Autodesk Fusion 360 part; units mm, degrees
note: some values were not read from the file. Set by a fixed rule: which sketch regions a step uses.
(part 2 of 4)
sketch "スケッチ25" plane through (0, 0, 3) normal (0, 0, 1) x (-1, 0, 0)
  line L0 (26.0567, 42.6737) -> (45.0073, 61.6244)
  line L1 (45.0073, 61.6244) -> (61.6244, 45.0073)
  line L2 (61.6244, 45.0073) -> (42.6737, 26.0567)
  arc A0 (42.6737, 26.0567) -> (26.0567, 42.6737) centre (0, 0) ccw
  line L3 (-36.2136, -34.4757) -> (-59.4233, -47.8758)
  line L4 (-59.4233, -47.8758) -> (-71.1733, -27.5242)
  line L5 (-71.1733, -27.5242) -> (-47.9636, -14.1241)
  arc A1 (-47.9636, -14.1241) -> (-36.2136, -34.4757) centre (0, 0) ccw
  arc A2 (-32.4242, -38.0614) -> (-21.7945, -45) centre (0, 0) ccw
  line L6 (-21.7945, -45) -> (-44.4423, -45)
  line L7 (-44.4423, -45) -> (-32.4242, -38.0614)
  line L8 (81.8683, -9) -> (73.6733, -23.1941)
  line L9 (73.6733, -23.1941) -> (49.1742, -9.0495)
  line L10 (49.1742, -9.0495) -> (75, -9)
  line L11 (75, -9) -> (81.8683, -9)
  line L12 (-42.6737, 26.0567) -> (-61.6244, 45.0073)
  line L13 (-61.6244, 45.0073) -> (-45.0073, 61.6244)
  line L14 (-45.0073, 61.6244) -> (-26.0567, 42.6737)
  arc A3 (-26.0567, 42.6737) -> (-42.6737, 26.0567) centre (0, 0) ccw
  line L15 (47.9636, -14.1241) -> (71.1733, -27.5242)
  line L16 (71.1733, -27.5242) -> (59.4233, -47.8758)
  line L17 (59.4233, -47.8758) -> (36.2136, -34.4757)
  arc A4 (36.2136, -34.4757) -> (47.9636, -14.1241) centre (0, 0) ccw
  line L18 (-81.8759, -8.9868) -> (-49.1742, -9.0495)
  line L19 (-49.1742, -9.0495) -> (-73.6733, -23.1941)
  line L20 (-73.6733, -23.1941) -> (-81.8759, -8.9868)
  line L21 (32.4242, -38.0614) -> (44.4423, -45)
  line L22 (44.4423, -45) -> (21.7945, -45)
  arc A5 (21.7945, -45) -> (32.4242, -38.0614) centre (0, 0) ccw
  arc A6 (44.8219, 4) -> (33.996, 29.4834) centre (0, 0) ccw
  line L23 (44.8219, 4) -> (98.9192, 4)
  arc A7 (98.9192, -4) -> (98.9192, 4) centre (0, 0) ccw
  line L24 (98.9192, -4) -> (44.8219, -4)
  arc A8 (33.0729, -30.5153) -> (44.8219, -4) centre (0, 0) ccw
  line L25 (33.0729, -30.5153) -> (27.4933, -24.7612)
  arc A9 (27.4933, -24.7612) -> (28.242, 23.9038) centre (0, 0) ccw
  line L26 (28.242, 23.9038) -> (33.996, 29.4834)
  arc A10 (4, -44.8219) -> (29.4834, -33.996) centre (0, 0) ccw
  line L27 (4, -44.8219) -> (4, -50)
  line L28 (4, -50) -> (40, -50)
  line L29 (40, -50) -> (40, -58)
  line L30 (40, -58) -> (-40, -58)
  line L31 (-40, -58) -> (-40, -50)
  line L32 (-40, -50) -> (-4, -50)
  line L33 (-4, -50) -> (-4, -47)
  line L34 (-4, -47) -> (-4, -44.8219)
  arc A11 (-30.5153, -33.0729) -> (-4, -44.8219) centre (0, 0) ccw
  line L35 (-30.5153, -33.0729) -> (-24.7612, -27.4933)
  arc A12 (-24.7612, -27.4933) -> (23.9038, -28.242) centre (0, 0) ccw
  line L36 (23.9038, -28.242) -> (29.4834, -33.996)
  line L37 (30.5153, 33.0729) -> (24.7612, 27.4933)
  arc A13 (24.7612, 27.4933) -> (-23.9038, 28.242) centre (0, 0) ccw
  line L38 (-23.9038, 28.242) -> (-29.4834, 33.996)
  arc A14 (-4, 44.8219) -> (-29.4834, 33.996) centre (0, 0) ccw
  line L39 (-4, 44.8219) -> (-4, 98.9192)
  arc A15 (4, 98.9192) -> (-4, 98.9192) centre (0, 0) ccw
  line L40 (4, 98.9192) -> (4, 44.8219)
  arc A16 (30.5153, 33.0729) -> (4, 44.8219) centre (0, 0) ccw
  circle A17 centre (0, 0) radius 32
  line L41 (-33.0729, 30.5153) -> (-27.4933, 24.7612)
  arc A18 (-27.4933, 24.7612) -> (-28.242, -23.9038) centre (0, 0) ccw
  line L42 (-28.242, -23.9038) -> (-33.996, -29.4834)
  arc A19 (-44.8219, -4) -> (-33.996, -29.4834) centre (0, 0) ccw
  line L43 (-44.8219, -4) -> (-98.9192, -4)
  arc A20 (-98.9192, 4) -> (-98.9192, -4) centre (0, 0) ccw
  line L44 (-98.9192, 4) -> (-44.8219, 4)
  arc A21 (-33.0729, 30.5153) -> (-44.8219, 4) centre (0, 0) ccw
  circle A22 centre (-51.2451, -46.0409) radius 1.5
  circle A23 centre (51.2451, -46.0409) radius 1.5
  circle A24 centre (-65.4951, -21.3591) radius 1.5
  circle A25 centre (-57.7353, 37.5827) radius 1.5
  circle A26 centre (-37.5827, 57.7353) radius 1.5
  circle A27 centre (37.5827, 57.7353) radius 1.5
  circle A28 centre (57.7353, 37.5827) radius 1.5
  circle A29 centre (65.4951, -21.3591) radius 1.5
  line L45 (40, -84.2208) -> (61.0153, -84.2208)
  arc A30 (61.0153, -84.2208) -> (71.238, -75.7703) centre (0, 0) ccw
  line L46 (71.238, -75.7703) -> (54.6284, -66.1808)
  line L47 (54.6284, -66.1808) -> (84.6284, -14.2192)
  line L48 (84.6284, -14.2192) -> (101.238, -23.8088)
  arc A31 (101.238, -23.8088) -> (91.6263, 49.1999) centre (0, 0) ccw
  line L49 (91.6263, 49.1999) -> (78.0646, 35.6382)
  line L50 (78.0646, 35.6382) -> (35.6382, 78.0646)
  line L51 (35.6382, 78.0646) -> (49.1999, 91.6263)
  arc A32 (49.1999, 91.6263) -> (-49.1999, 91.6263) centre (0, 0) ccw
  line L52 (-49.1999, 91.6263) -> (-35.6382, 78.0646)
  line L53 (-35.6382, 78.0646) -> (-78.0646, 35.6382)
  line L54 (-78.0646, 35.6382) -> (-91.6263, 49.1999)
  arc A33 (-91.6263, 49.1999) -> (-101.238, -23.8088) centre (0, 0) ccw
  line L55 (-101.238, -23.8088) -> (-84.6284, -14.2192)
  line L56 (-84.6284, -14.2192) -> (-54.6284, -66.1808)
  line L57 (-54.6284, -66.1808) -> (-71.238, -75.7703)
  arc A34 (-71.238, -75.7703) -> (-61.3188, -84) centre (0, 0) ccw
  line L58 (-61.3188, -84) -> (-40, -84)
  line L59 (-40, -84) -> (-40, -64)
  line L60 (-40, -64) -> (40, -64)
  line L61 (40, -64) -> (40, -84.2208)
  line L62 (0, 0) -> (-27.7575, -27.7575)
  line L63 (0, 0) -> (39.2551, 0) construction
  line L64 (-27.7575, -27.7575) -> (-26.0172, -29.5523)
  line L65 (-26.0172, -29.5523) -> (-30.0678, -33.4802)
  line L66 (-26.0172, -29.5523) -> (-24.308, -27.8949)
  line L67 (0, 0) -> (31.8198, -31.8198)
  line L68 (0, 0) -> (45, 0) construction
  line L69 (0, 0) -> (-34.0048, 34.0048)
  line L70 (0, 0) -> (29.8779, 29.8779)
  line L71 (-27.7575, -27.7575) -> (-26.0172, -29.5523)
  line L72 (-26.0172, -29.5523) -> (-24.308, -27.8949)
  line L73 (-26.0172, -29.5523) -> (-30.0678, -33.4802)
  line L74 (29.2, -29.2) -> (30.9678, -27.4322)
  line L75 (30.9678, -27.4322) -> (33.5384, -30.0029)
  line L76 (30.9678, -27.4322) -> (27.8709, -24.3354)
  line L77 (29.8779, 29.8779) -> (28.1102, 31.6457)
  line L78 (28.1102, 31.6457) -> (30.0029, 33.5384)
  line L79 (28.1102, 31.6457) -> (24.3354, 27.8709)
  line L80 (-29.5, 29.5) -> (-31.2948, 27.7596)
  line L81 (-31.2948, 27.7596) -> (-27.9198, 24.2793)
  line L82 (-31.2948, 27.7596) -> (-33.5056, 30.0396)
  dimension "d100" = 135
  dimension "d101" = 2.5
  dimension "d102" = 45
  dimension "d103" = 45
  dimension "d104" = 2.5
  dimension "d105" = 2.5
  dimension "d106" = 2.5
  constraint horizontal L63
  constraint coincident A0.centre A1.centre
  constraint perpendicular L35 L64
  constraint coincident A11 L65.end
  constraint perpendicular L64 L65
  constraint coincident A12 L66.end
  constraint perpendicular L64 L66
  constraint horizontal L68
  constraint parallel L67 L69
  constraint perpendicular L69 L70
  constraint coincident L67 L74.start
  constraint perpendicular L67 L74
  constraint coincident A8 L75.end
  constraint perpendicular L74 L75
  constraint coincident A9 L76.end
  constraint perpendicular L74 L76
  constraint perpendicular L70 L77
  constraint coincident A16 L78.end
  constraint perpendicular L77 L78
  constraint coincident A13 L79.end
  constraint perpendicular L77 L79
  constraint coincident L69 L80.start
  constraint perpendicular L41 L80
  constraint coincident A18 L81.end
  constraint perpendicular L80 L81
  constraint coincident A21 L82.end
  constraint perpendicular L80 L82
  measures "d100" angle of L62 L63
  measures "d101" distance of L62.end L64.end
  measures "d102" distance of A0.centre L67.end
  measures "d103" angle of L67 L68
  measures "d104" distance of L74.start L74.end
  measures "d105" distance of L70.end L77.end
  measures "d106" distance of L80.start L80.end
extrude "押し出し24" add sketch "スケッチ25" against normal blind 1.5 contours L25 A9 L74 L76 | A8 L25 L74 L75 | L35 A12 L64 L66 L71 L72 | A11 L35 L64 L65 L71 L73 | L37 A16 L77 L78 | L37 A13 L77 L79 | L41 A21 L80 L82 | L41 A18 L80 L81 bodies 1
sketch "スケッチ26" plane through (0, 0, 3) normal (0, 0, 1) x (-1, 0, 0)
  line L0 (26.0567, 42.6737) -> (45.0073, 61.6244)
  line L1 (45.0073, 61.6244) -> (61.6244, 45.0073)
  line L2 (61.6244, 45.0073) -> (42.6737, 26.0567)
  arc A0 (42.6737, 26.0567) -> (26.0567, 42.6737) centre (0, 0) ccw
  line L3 (-36.2136, -34.4757) -> (-59.4233, -47.8758)
  line L4 (-59.4233, -47.8758) -> (-71.1733, -27.5242)
  line L5 (-71.1733, -27.5242) -> (-47.9636, -14.1241)
  arc A1 (-47.9636, -14.1241) -> (-36.2136, -34.4757) centre (0, 0) ccw
  arc A2 (-32.4242, -38.0614) -> (-21.7945, -45) centre (0, 0) ccw
  line L6 (-21.7945, -45) -> (-44.4423, -45)
  line L7 (-44.4423, -45) -> (-32.4242, -38.0614)
  line L8 (81.8683, -9) -> (73.6733, -23.1941)
  line L9 (73.6733, -23.1941) -> (49.1742, -9.0495)
  line L10 (49.1742, -9.0495) -> (75, -9)
  line L11 (75, -9) -> (81.8683, -9)
  line L12 (-42.6737, 26.0567) -> (-61.6244, 45.0073)
  line L13 (-61.6244, 45.0073) -> (-45.0073, 61.6244)
  line L14 (-45.0073, 61.6244) -> (-26.0567, 42.6737)
  arc A3 (-26.0567, 42.6737) -> (-42.6737, 26.0567) centre (0, 0) ccw
  line L15 (47.9636, -14.1241) -> (71.1733, -27.5242)
  line L16 (71.1733, -27.5242) -> (59.4233, -47.8758)
  line L17 (59.4233, -47.8758) -> (36.2136, -34.4757)
  arc A4 (36.2136, -34.4757) -> (47.9636, -14.1241) centre (0, 0) ccw
  line L18 (-81.8759, -8.9868) -> (-49.1742, -9.0495)
  line L19 (-49.1742, -9.0495) -> (-73.6733, -23.1941)
  line L20 (-73.6733, -23.1941) -> (-81.8759, -8.9868)
  line L21 (32.4242, -38.0614) -> (44.4423, -45)
  line L22 (44.4423, -45) -> (21.7945, -45)
  arc A5 (21.7945, -45) -> (32.4242, -38.0614) centre (0, 0) ccw
  arc A6 (44.8219, 4) -> (33.996, 29.4834) centre (0, 0) ccw
  line L23 (44.8219, 4) -> (98.9192, 4)
  arc A7 (98.9192, -4) -> (98.9192, 4) centre (0, 0) ccw
  line L24 (98.9192, -4) -> (44.8219, -4)
  arc A8 (33.5384, -30.0029) -> (44.8219, -4) centre (0, 0) ccw
  line L25 (33.5384, -30.0029) -> (27.8709, -24.3354)
  arc A9 (27.8709, -24.3354) -> (28.242, 23.9038) centre (0, 0) ccw
  line L26 (28.242, 23.9038) -> (33.996, 29.4834)
  arc A10 (4, -44.8219) -> (29.4834, -33.996) centre (0, 0) ccw
  line L27 (4, -44.8219) -> (4, -50)
  line L28 (4, -50) -> (40, -50)
  line L29 (40, -50) -> (40, -58)
  line L30 (40, -58) -> (-40, -58)
  line L31 (-40, -58) -> (-40, -50)
  line L32 (-40, -50) -> (-4, -50)
  line L33 (-4, -50) -> (-4, -47)
  line L34 (-4, -47) -> (-4, -44.8219)
  arc A11 (-30.0678, -33.4802) -> (-4, -44.8219) centre (0, 0) ccw
  line L35 (-30.0678, -33.4802) -> (-24.308, -27.8949)
  arc A12 (-24.308, -27.8949) -> (23.9038, -28.242) centre (0, 0) ccw
  line L36 (23.9038, -28.242) -> (29.4834, -33.996)
  arc A13 (24.3354, 27.8709) -> (-23.9038, 28.242) centre (0, 0) ccw
  line L37 (-23.9038, 28.242) -> (-29.4834, 33.996)
  arc A14 (-4, 44.8219) -> (-29.4834, 33.996) centre (0, 0) ccw
  line L38 (-4, 44.8219) -> (-4, 98.9192)
  arc A15 (4, 98.9192) -> (-4, 98.9192) centre (0, 0) ccw
  line L39 (4, 98.9192) -> (4, 44.8219)
  arc A16 (30.0029, 33.5384) -> (4, 44.8219) centre (0, 0) ccw
  line L40 (30.0029, 33.5384) -> (24.3354, 27.8709)
  circle A17 centre (0, 0) radius 32
  arc A18 (-27.9198, 24.2793) -> (-28.242, -23.9038) centre (0, 0) ccw
  line L41 (-28.242, -23.9038) -> (-33.996, -29.4834)
  arc A19 (-44.8219, -4) -> (-33.996, -29.4834) centre (0, 0) ccw
  line L42 (-44.8219, -4) -> (-98.9192, -4)
  arc A20 (-98.9192, 4) -> (-98.9192, -4) centre (0, 0) ccw
  line L43 (-98.9192, 4) -> (-44.8219, 4)
  arc A21 (-33.5056, 30.0396) -> (-44.8219, 4) centre (0, 0) ccw
  line L44 (-33.5056, 30.0396) -> (-27.9198, 24.2793)
  circle A22 centre (-51.2451, -46.0409) radius 1.5
  circle A23 centre (51.2451, -46.0409) radius 1.5
  circle A24 centre (-65.4951, -21.3591) radius 1.5
  circle A25 centre (-57.7353, 37.5827) radius 1.5
  circle A26 centre (-37.5827, 57.7353) radius 1.5
  circle A27 centre (37.5827, 57.7353) radius 1.5
  circle A28 centre (57.7353, 37.5827) radius 1.5
  circle A29 centre (65.4951, -21.3591) radius 1.5
  line L45 (40, -84.2208) -> (61.0153, -84.2208)
  arc A30 (61.0153, -84.2208) -> (71.238, -75.7703) centre (0, 0) ccw
  line L46 (71.238, -75.7703) -> (54.6284, -66.1808)
  line L47 (54.6284, -66.1808) -> (84.6284, -14.2192)
  line L48 (84.6284, -14.2192) -> (101.238, -23.8088)
  arc A31 (101.238, -23.8088) -> (91.6263, 49.1999) centre (0, 0) ccw
  line L49 (91.6263, 49.1999) -> (78.0646, 35.6382)
  line L50 (78.0646, 35.6382) -> (35.6382, 78.0646)
  line L51 (35.6382, 78.0646) -> (49.1999, 91.6263)
  arc A32 (49.1999, 91.6263) -> (-49.1999, 91.6263) centre (0, 0) ccw
  line L52 (-49.1999, 91.6263) -> (-35.6382, 78.0646)
  line L53 (-35.6382, 78.0646) -> (-78.0646, 35.6382)
  line L54 (-78.0646, 35.6382) -> (-91.6263, 49.1999)
  arc A33 (-91.6263, 49.1999) -> (-101.238, -23.8088) centre (0, 0) ccw
  line L55 (-101.238, -23.8088) -> (-84.6284, -14.2192)
  line L56 (-84.6284, -14.2192) -> (-54.6284, -66.1808)
  line L57 (-54.6284, -66.1808) -> (-71.238, -75.7703)
  arc A34 (-71.238, -75.7703) -> (-61.3188, -84) centre (0, 0) ccw
  line L58 (-61.3188, -84) -> (-40, -84)
  line L59 (-40, -84) -> (-40, -64)
  line L60 (-40, -64) -> (40, -64)
  line L61 (40, -64) -> (40, -84.2208)
  line L62 (0, 0) -> (33.4792, -33.4792)
  line L63 (0, 0) -> (47.3468, 0) construction
  line L64 (0, 0) -> (-28.242, -28.242)
  line L65 (0, 0) -> (-27.5799, 27.5799)
  line L66 (0, 0) -> (30, 30)
  line L67 (29, -29) -> (27.2322, -30.7678)
  line L68 (-27.6978, -27.6978) -> (-29.4655, -25.93)
  line L69 (-27, 27) -> (-25.2322, 28.7678)
  line L70 (28, 28) -> (29.7678, 26.2322)
  circle A35 centre (0, 0) radius 37
  circle A36 centre (0, 0) radius 45
  line L71 (29.7678, 26.2322) -> (27.8709, 24.3354)
  line L72 (29.7678, 26.2322) -> (33.5384, 30.0029)
  line L73 (-25.2322, 28.7678) -> (-24.3354, 27.8709)
  line L74 (-25.2322, 28.7678) -> (-30.0029, 33.5384)
  line L75 (-29.4655, -25.93) -> (-27.8709, -24.3354)
  line L76 (-29.4655, -25.93) -> (-33.5384, -30.0029)
  line L77 (27.2322, -30.7678) -> (24.3354, -27.8709)
  line L78 (27.2322, -30.7678) -> (30.0029, -33.5384)
  dimension "d109" = 45
  dimension "d110" = 2.5
  dimension "d111" = 2.5
  dimension "d112" = 2.5
  dimension "d113" = 2.5
  constraint horizontal L63
  constraint coincident A0.centre A1.centre
  constraint perpendicular L62 L64
  constraint perpendicular L64 L65
  constraint perpendicular L65 L66
  constraint coincident L62 L67.start
  constraint perpendicular L62 L67
  constraint coincident L64 L68.start
  constraint perpendicular L64 L68
  constraint coincident L65 L69.start
  constraint perpendicular L65 L69
  constraint coincident L66 L70.start
  constraint perpendicular L66 L70
  constraint coincident A35 L71.end
  constraint perpendicular L70 L71
  constraint coincident A36 L72.end
  constraint perpendicular L70 L72
  constraint coincident A35 L73.end
  constraint perpendicular L69 L73
  constraint coincident A36 L74.end
  constraint perpendicular L69 L74
  constraint coincident A35 L75.end
  constraint perpendicular L68 L75
  constraint coincident A36 L76.end
  constraint perpendicular L68 L76
  constraint coincident A35 L77.end
  constraint perpendicular L67 L77
  constraint coincident A36 L78.end
  constraint perpendicular L67 L78
  measures "d109" angle of L62 L63
  measures "d110" distance of L67.start L67.end
  measures "d111" distance of L68.start L68.end
  measures "d112" distance of L69.start L69.end
  measures "d113" distance of L70.start L70.end
extrude "押し出し25" cut sketch "スケッチ26" against normal blind 3.5 contours L26 A35 A36 L71 L72 | L37 A35 A36 L73 L74 | L36 A35 A36 L77 L78 | L41 A35 A36 L75 L76 bodies 1
sketch "スケッチ27" plane through (0, 0, 3) normal (0, 0, 1) x (-1, 0, 0)
  arc A0 (-4, 44.8219) -> (-30.0029, 33.5384) centre (0, 0) ccw
  line L0 (-4, 44.8219) -> (-4, 98.9192)
  arc A1 (4, 98.9192) -> (-4, 98.9192) centre (0, 0) ccw
  line L1 (4, 98.9192) -> (4, 44.8219)
  arc A2 (30.0029, 33.5384) -> (4, 44.8219) centre (0, 0) ccw
  line L2 (30.0029, 33.5384) -> (24.3354, 27.8709)
  arc A3 (24.3354, 27.8709) -> (-24.3354, 27.8709) centre (0, 0) ccw
  line L3 (-24.3354, 27.8709) -> (-30.0029, 33.5384)
  arc A4 (-44.8219, -4) -> (-33.5384, -30.0029) centre (0, 0) ccw
  line L4 (-44.8219, -4) -> (-98.9192, -4)
  arc A5 (-98.9192, 4) -> (-98.9192, -4) centre (0, 0) ccw
  line L5 (-98.9192, 4) -> (-44.8219, 4)
  arc A6 (-33.5056, 30.0396) -> (-44.8219, 4) centre (0, 0) ccw
  line L6 (-33.5056, 30.0396) -> (-27.9198, 24.2793)
  arc A7 (-27.9198, 24.2793) -> (-27.8709, -24.3354) centre (0, 0) ccw
  line L7 (-27.8709, -24.3354) -> (-33.5384, -30.0029)
  arc A8 (44.8219, 4) -> (33.5384, 30.0029) centre (0, 0) ccw
  line L8 (44.8219, 4) -> (98.9192, 4)
  arc A9 (98.9192, -4) -> (98.9192, 4) centre (0, 0) ccw
  line L9 (98.9192, -4) -> (44.8219, -4)
  arc A10 (33.5384, -30.0029) -> (44.8219, -4) centre (0, 0) ccw
  line L10 (33.5384, -30.0029) -> (27.8709, -24.3354)
  arc A11 (27.8709, -24.3354) -> (27.8709, 24.3354) centre (0, 0) ccw
  line L11 (27.8709, 24.3354) -> (33.5384, 30.0029)
  arc A12 (4, -44.8219) -> (30.0029, -33.5384) centre (0, 0) ccw
  line L12 (4, -44.8219) -> (4, -50)
  line L13 (4, -50) -> (40, -50)
  line L14 (40, -50) -> (40, -58)
  line L15 (40, -58) -> (-40, -58)
  line L16 (-40, -58) -> (-40, -50)
  line L17 (-40, -50) -> (-4, -50)
  line L18 (-4, -50) -> (-4, -47)
  line L19 (-4, -47) -> (-4, -44.8219)
  arc A13 (-30.0678, -33.4802) -> (-4, -44.8219) centre (0, 0) ccw
  line L20 (-30.0678, -33.4802) -> (-24.308, -27.8949)
  arc A14 (-24.308, -27.8949) -> (24.3354, -27.8709) centre (0, 0) ccw
  line L21 (24.3354, -27.8709) -> (30.0029, -33.5384)
  line L22 (26.0567, 42.6737) -> (45.0073, 61.6244)
  line L23 (45.0073, 61.6244) -> (61.6244, 45.0073)
  line L24 (61.6244, 45.0073) -> (42.6737, 26.0567)
  arc A15 (42.6737, 26.0567) -> (26.0567, 42.6737) centre (0, 0) ccw
  line L25 (-36.2136, -34.4757) -> (-59.4233, -47.8758)
  line L26 (-59.4233, -47.8758) -> (-71.1733, -27.5242)
  line L27 (-71.1733, -27.5242) -> (-47.9636, -14.1241)
  arc A16 (-47.9636, -14.1241) -> (-36.2136, -34.4757) centre (0, 0) ccw
  arc A17 (-32.4242, -38.0614) -> (-21.7945, -45) centre (0, 0) ccw
  line L28 (-21.7945, -45) -> (-44.4423, -45)
  line L29 (-44.4423, -45) -> (-32.4242, -38.0614)
  line L30 (81.8683, -9) -> (73.6733, -23.1941)
  line L31 (73.6733, -23.1941) -> (49.1742, -9.0495)
  line L32 (49.1742, -9.0495) -> (75, -9)
  line L33 (75, -9) -> (81.8683, -9)
  line L34 (-42.6737, 26.0567) -> (-61.6244, 45.0073)
  line L35 (-61.6244, 45.0073) -> (-45.0073, 61.6244)
  line L36 (-45.0073, 61.6244) -> (-26.0567, 42.6737)
  arc A18 (-26.0567, 42.6737) -> (-42.6737, 26.0567) centre (0, 0) ccw
  line L37 (47.9636, -14.1241) -> (71.1733, -27.5242)
  line L38 (71.1733, -27.5242) -> (59.4233, -47.8758)
  line L39 (59.4233, -47.8758) -> (36.2136, -34.4757)
  arc A19 (36.2136, -34.4757) -> (47.9636, -14.1241) centre (0, 0) ccw
  line L40 (-81.8759, -8.9868) -> (-49.1742, -9.0495)
  line L41 (-49.1742, -9.0495) -> (-73.6733, -23.1941)
  line L42 (-73.6733, -23.1941) -> (-81.8759, -8.9868)
  line L43 (32.4242, -38.0614) -> (44.4423, -45)
  line L44 (44.4423, -45) -> (21.7945, -45)
  arc A20 (21.7945, -45) -> (32.4242, -38.0614) centre (0, 0) ccw
  circle A21 centre (0, 0) radius 32
  circle A22 centre (-51.2451, -46.0409) radius 1.5
  circle A23 centre (51.2451, -46.0409) radius 1.5
  circle A24 centre (-65.4951, -21.3591) radius 1.5
  circle A25 centre (-57.7353, 37.5827) radius 1.5
  circle A26 centre (-37.5827, 57.7353) radius 1.5
  circle A27 centre (37.5827, 57.7353) radius 1.5
  circle A28 centre (57.7353, 37.5827) radius 1.5
  circle A29 centre (65.4951, -21.3591) radius 1.5
  line L45 (40, -84.2208) -> (61.0153, -84.2208)
  arc A30 (61.0153, -84.2208) -> (71.238, -75.7703) centre (0, 0) ccw
  line L46 (71.238, -75.7703) -> (54.6284, -66.1808)
  line L47 (54.6284, -66.1808) -> (84.6284, -14.2192)
  line L48 (84.6284, -14.2192) -> (101.238, -23.8088)
  arc A31 (101.238, -23.8088) -> (91.6263, 49.1999) centre (0, 0) ccw
  line L49 (91.6263, 49.1999) -> (78.0646, 35.6382)
  line L50 (78.0646, 35.6382) -> (35.6382, 78.0646)
  line L51 (35.6382, 78.0646) -> (49.1999, 91.6263)
  arc A32 (49.1999, 91.6263) -> (-49.1999, 91.6263) centre (0, 0) ccw
  line L52 (-49.1999, 91.6263) -> (-35.6382, 78.0646)
  line L53 (-35.6382, 78.0646) -> (-78.0646, 35.6382)
  line L54 (-78.0646, 35.6382) -> (-91.6263, 49.1999)
  arc A33 (-91.6263, 49.1999) -> (-101.238, -23.8088) centre (0, 0) ccw
  line L55 (-101.238, -23.8088) -> (-84.6284, -14.2192)
  line L56 (-84.6284, -14.2192) -> (-54.6284, -66.1808)
  line L57 (-54.6284, -66.1808) -> (-71.238, -75.7703)
  arc A34 (-71.238, -75.7703) -> (-61.3188, -84) centre (0, 0) ccw
  line L58 (-61.3188, -84) -> (-40, -84)
  line L59 (-40, -84) -> (-40, -64)
  line L60 (-40, -64) -> (40, -64)
  line L61 (40, -64) -> (40, -84.2208)
  circle A35 centre (0, 0) radius 99
  line L62 (-90, -4) -> (-90, -9.0182)
  line L63 (-90, -9.0182) -> (-98.5884, -9.0182)
  line L64 (-92.9332, -19.014) -> (-95.4332, -14.6839)
  line L65 (-95.4332, -14.6839) -> (-97.6998, -15.9925)
  line L66 (-95.4332, -14.6839) -> (-85.6199, -9.0182)
  line L67 (-85.6199, -9.0182) -> (-90, -9.0182)
  line L68 (92.9332, -19.014) -> (95.4332, -14.6839)
  line L69 (95.4332, -14.6839) -> (97.6998, -15.9925)
  line L70 (93, -4) -> (93, -9.0182)
  line L71 (93, -9.0182) -> (98.5884, -9.0182)
  line L72 (95.4332, -14.6839) -> (85.6199, -9.0182)
  line L73 (85.6199, -9.0182) -> (93, -9.0182)
  dimension "d116" = 5
  dimension "d117" = 5
  constraint coincident A0.centre A1.centre
  constraint coincident L4 L62.start
  constraint perpendicular L4 L62
  constraint coincident A35 L63.end
  constraint perpendicular L62 L63
  constraint midpoint L55 L64.start
  constraint perpendicular L55 L64
  constraint coincident A35 L65.end
  constraint perpendicular L64 L65
  constraint perpendicular L64 L66
  constraint perpendicular L62 L67
  constraint midpoint L48 L68.start
  constraint perpendicular L48 L68
  constraint coincident A35 L69.end
  constraint perpendicular L30 L69
  constraint coincident L9 L70.start
  constraint perpendicular L9 L70
  constraint coincident A35 L71.end
  constraint perpendicular L70 L71
  constraint perpendicular L68 L72
  constraint perpendicular L70 L73
  measures "d116" distance of L64.start L64.end
  measures "d117" distance of L68.start L68.end
extrude "押し出し26" cut sketch "スケッチ27" against normal blind 25 contours A35 L63 L65 L66 L67 | A35 L69 L71 L72 L73 bodies 1
sketch "スケッチ28" plane through (0, 0, 3) normal (0, 0, 1) x (-1, 0, 0)
  arc A0 (97.6998, -15.9925) -> (98.5884, -9.0182) centre (0, 0) ccw
  line L0 (97.6998, -15.9925) -> (85.6199, -9.0182)
  line L1 (85.6199, -9.0182) -> (98.5884, -9.0182)
  line L2 (-98.5884, -9.0182) -> (-85.6199, -9.0182)
  line L3 (-85.6199, -9.0182) -> (-97.6998, -15.9925)
  arc A1 (-98.5884, -9.0182) -> (-97.6998, -15.9925) centre (0, 0) ccw
  arc A2 (-4, 44.8219) -> (-30.0029, 33.5384) centre (0, 0) ccw
  line L4 (-4, 44.8219) -> (-4, 98.9192)
  arc A3 (4, 98.9192) -> (-4, 98.9192) centre (0, 0) ccw
  line L5 (4, 98.9192) -> (4, 44.8219)
  arc A4 (30.0029, 33.5384) -> (4, 44.8219) centre (0, 0) ccw
  line L6 (30.0029, 33.5384) -> (24.3354, 27.8709)
  arc A5 (24.3354, 27.8709) -> (-24.3354, 27.8709) centre (0, 0) ccw
  line L7 (-24.3354, 27.8709) -> (-30.0029, 33.5384)
  arc A6 (-44.8219, -4) -> (-33.5384, -30.0029) centre (0, 0) ccw
  line L8 (-44.8219, -4) -> (-98.9192, -4)
  arc A7 (-98.9192, 4) -> (-98.9192, -4) centre (0, 0) ccw
  line L9 (-98.9192, 4) -> (-44.8219, 4)
  arc A8 (-33.5056, 30.0396) -> (-44.8219, 4) centre (0, 0) ccw
  line L10 (-33.5056, 30.0396) -> (-27.9198, 24.2793)
  arc A9 (-27.9198, 24.2793) -> (-27.8709, -24.3354) centre (0, 0) ccw
  line L11 (-27.8709, -24.3354) -> (-33.5384, -30.0029)
  arc A10 (44.8219, 4) -> (33.5384, 30.0029) centre (0, 0) ccw
  line L12 (44.8219, 4) -> (98.9192, 4)
  arc A11 (98.9192, -4) -> (98.9192, 4) centre (0, 0) ccw
  line L13 (98.9192, -4) -> (44.8219, -4)
  arc A12 (33.5384, -30.0029) -> (44.8219, -4) centre (0, 0) ccw
  line L14 (33.5384, -30.0029) -> (27.8709, -24.3354)
  arc A13 (27.8709, -24.3354) -> (27.8709, 24.3354) centre (0, 0) ccw
  line L15 (27.8709, 24.3354) -> (33.5384, 30.0029)
  arc A14 (4, -44.8219) -> (30.0029, -33.5384) centre (0, 0) ccw
  line L16 (4, -44.8219) -> (4, -50)
  line L17 (4, -50) -> (40, -50)
  line L18 (40, -50) -> (40, -58)
  line L19 (40, -58) -> (-40, -58)
  line L20 (-40, -58) -> (-40, -50)
  line L21 (-40, -50) -> (-4, -50)
  line L22 (-4, -50) -> (-4, -47)
  line L23 (-4, -47) -> (-4, -44.8219)
  arc A15 (-30.0678, -33.4802) -> (-4, -44.8219) centre (0, 0) ccw
  line L24 (-30.0678, -33.4802) -> (-24.308, -27.8949)
  arc A16 (-24.308, -27.8949) -> (24.3354, -27.8709) centre (0, 0) ccw
  line L25 (24.3354, -27.8709) -> (30.0029, -33.5384)
  line L26 (26.0567, 42.6737) -> (45.0073, 61.6244)
  line L27 (45.0073, 61.6244) -> (61.6244, 45.0073)
  line L28 (61.6244, 45.0073) -> (42.6737, 26.0567)
  arc A17 (42.6737, 26.0567) -> (26.0567, 42.6737) centre (0, 0) ccw
  line L29 (-36.2136, -34.4757) -> (-59.4233, -47.8758)
  line L30 (-59.4233, -47.8758) -> (-71.1733, -27.5242)
  line L31 (-71.1733, -27.5242) -> (-47.9636, -14.1241)
  arc A18 (-47.9636, -14.1241) -> (-36.2136, -34.4757) centre (0, 0) ccw
  arc A19 (-32.4242, -38.0614) -> (-21.7945, -45) centre (0, 0) ccw
  line L32 (-21.7945, -45) -> (-44.4423, -45)
  line L33 (-44.4423, -45) -> (-32.4242, -38.0614)
  line L34 (81.8683, -9) -> (73.6733, -23.1941)
  line L35 (73.6733, -23.1941) -> (49.1742, -9.0495)
  line L36 (49.1742, -9.0495) -> (75, -9)
  line L37 (75, -9) -> (81.8683, -9)
  line L38 (-42.6737, 26.0567) -> (-61.6244, 45.0073)
  line L39 (-61.6244, 45.0073) -> (-45.0073, 61.6244)
  line L40 (-45.0073, 61.6244) -> (-26.0567, 42.6737)
  arc A20 (-26.0567, 42.6737) -> (-42.6737, 26.0567) centre (0, 0) ccw
  line L41 (47.9636, -14.1241) -> (71.1733, -27.5242)
  line L42 (71.1733, -27.5242) -> (59.4233, -47.8758)
  line L43 (59.4233, -47.8758) -> (36.2136, -34.4757)
  arc A21 (36.2136, -34.4757) -> (47.9636, -14.1241) centre (0, 0) ccw
  line L44 (-81.8759, -8.9868) -> (-49.1742, -9.0495)
  line L45 (-49.1742, -9.0495) -> (-73.6733, -23.1941)
  line L46 (-73.6733, -23.1941) -> (-81.8759, -8.9868)
  line L47 (32.4242, -38.0614) -> (44.4423, -45)
  line L48 (44.4423, -45) -> (21.7945, -45)
  arc A22 (21.7945, -45) -> (32.4242, -38.0614) centre (0, 0) ccw
  circle A23 centre (0, 0) radius 32
  circle A24 centre (-51.2451, -46.0409) radius 1.5
  circle A25 centre (51.2451, -46.0409) radius 1.5
  circle A26 centre (-65.4951, -21.3591) radius 1.5
  circle A27 centre (-57.7353, 37.5827) radius 1.5
  circle A28 centre (-37.5827, 57.7353) radius 1.5
  circle A29 centre (37.5827, 57.7353) radius 1.5
  circle A30 centre (57.7353, 37.5827) radius 1.5
  circle A31 centre (65.4951, -21.3591) radius 1.5
  line L49 (40, -84.2208) -> (61.0153, -84.2208)
  arc A32 (61.0153, -84.2208) -> (71.238, -75.7703) centre (0, 0) ccw
  line L50 (71.238, -75.7703) -> (54.6284, -66.1808)
  line L51 (54.6284, -66.1808) -> (84.6284, -14.2192)
  line L52 (84.6284, -14.2192) -> (101.238, -23.8088)
  arc A33 (101.238, -23.8088) -> (91.6263, 49.1999) centre (0, 0) ccw
  line L53 (91.6263, 49.1999) -> (78.0646, 35.6382)
  line L54 (78.0646, 35.6382) -> (35.6382, 78.0646)
  line L55 (35.6382, 78.0646) -> (49.1999, 91.6263)
  arc A34 (49.1999, 91.6263) -> (-49.1999, 91.6263) centre (0, 0) ccw
  line L56 (-49.1999, 91.6263) -> (-35.6382, 78.0646)
  line L57 (-35.6382, 78.0646) -> (-78.0646, 35.6382)
  line L58 (-78.0646, 35.6382) -> (-91.6263, 49.1999)
  arc A35 (-91.6263, 49.1999) -> (-101.238, -23.8088) centre (0, 0) ccw
  line L59 (-101.238, -23.8088) -> (-84.6284, -14.2192)
  line L60 (-84.6284, -14.2192) -> (-54.6284, -66.1808)
  line L61 (-54.6284, -66.1808) -> (-71.238, -75.7703)
  arc A36 (-71.238, -75.7703) -> (-61.3188, -84) centre (0, 0) ccw
  line L62 (-61.3188, -84) -> (-40, -84)
  line L63 (-40, -84) -> (-40, -64)
  line L64 (-40, -64) -> (40, -64)
  line L65 (40, -64) -> (40, -84.2208)
  circle A37 centre (0, 0) radius 50
  circle A38 centre (0, 0) radius 99
  line L66 (-75, 4) -> (-75, 9)
  line L67 (-75, 9) -> (-98.5901, 9)
  line L68 (-75, 9) -> (-49.1833, 9)
  line L69 (-49.1833, 9) -> (-49.177, 9)
  line L70 (-57.7353, 37.5827) -> (-55.9675, 39.3505)
  line L71 (-57.7353, 37.5827) -> (-59.503, 35.815)
  line L72 (-59.503, 35.815) -> (-45.1565, 21.4684)
  line L73 (-61.6244, 45.0073) -> (-77.99, 28.6417)
  line L74 (-59.503, 35.815) -> (-65.1599, 41.4718)
  line L75 (-82.4813, 40.0549) -> (-86.0169, 36.5194)
  line L76 (-86.0169, 36.5194) -> (-77.0338, 27.5363)
  line L77 (-77.99, 28.6417) -> (-78.0646, 28.5671)
  line L78 (-86.0169, 36.5194) -> (-90.2316, 40.7341)
  line L79 (75, 4) -> (75, 9)
  line L80 (75, 9) -> (49.1833, 9)
  line L81 (75, 9) -> (98.5901, 9)
  line L82 (98.5901, 9) -> (99, 9)
  line L83 (57.7353, 37.5827) -> (55.9675, 39.3505)
  line L84 (57.7353, 37.5827) -> (59.503, 35.815)
  line L85 (59.503, 35.815) -> (45.1565, 21.4684)
  line L86 (59.503, 35.815) -> (67.2867, 43.5986)
  line L87 (61.6244, 45.0073) -> (77.99, 28.6417)
  line L88 (83.4561, 41.0297) -> (86.9916, 37.4941)
  line L89 (86.9916, 37.4941) -> (74.768, 25.2705)
  line L90 (77.99, 28.6417) -> (78.0646, 28.5671)
  line L91 (86.9916, 37.4941) -> (90.2316, 40.7341)
  line L92 (-37.5827, 57.7353) -> (-35.815, 59.503)
  line L93 (-35.815, 59.503) -> (-21.4684, 45.1565)
  line L94 (-45.0073, 61.6244) -> (-24.9598, 81.6719)
  line L95 (-35.815, 59.503) -> (-41.4718, 65.1599)
  line L96 (-40.5337, 82.9601) -> (-36.9982, 86.4957)
  line L97 (-36.9982, 86.4957) -> (-28.5671, 78.0646)
  line L98 (-36.9982, 86.4957) -> (-40.7341, 90.2316)
  line L99 (45.0073, 61.6244) -> (26.904, 79.7277)
  line L100 (39.8537, 82.2801) -> (36.3182, 85.8157)
  line L101 (36.3182, 85.8157) -> (28.5671, 78.0646)
  line L102 (36.3182, 85.8157) -> (40.7341, 90.2316)
  line L103 (37.5827, 57.7353) -> (35.815, 59.503)
  line L104 (35.815, 59.503) -> (41.4718, 65.1599)
  line L105 (35.815, 59.503) -> (21.4684, 45.1565)
  line L106 (4, 68.4061) -> (9, 68.4061)
  line L107 (9, 68.4061) -> (9, 49.1833)
  line L108 (9, 68.4061) -> (9, 98.5901)
  line L109 (-4, 68.4061) -> (-9, 68.4061)
  line L110 (-9, 68.4061) -> (-9, 49.1833)
  line L111 (-9, 68.4061) -> (-9, 99)
  dimension "d120" = 2.5
  dimension "d121" = 5
  dimension "d122" = 2.5
  dimension "d123" = 5
  dimension "d124" = 2.5
  dimension "d125" = 5
  dimension "d126" = 5
  dimension "d127" = 2.5
  constraint coincident A0.centre A1.centre
  constraint concentric A0 A38
  constraint coincident L9 L66.start
  constraint perpendicular L9 L66
  constraint coincident A38 L67.end
  constraint perpendicular L66 L67
  constraint coincident A37 L68.end
  constraint perpendicular L66 L68
  constraint parallel L68 L69
  constraint coincident A27.centre L70.start
  constraint coincident L38 L70.end
  constraint perpendicular L38 L70
  constraint perpendicular L38 L71
  constraint coincident A37 L72.end
  constraint perpendicular L71 L72
  constraint coincident L38.end L39.start
  constraint perpendicular L38 L73
  constraint coincident L73 L74.end
  constraint perpendicular L73 L74
  constraint coincident L58 L75.start
  constraint perpendicular L58 L75
  constraint perpendicular L73 L76
  constraint coincident L76 L77.end
  constraint perpendicular L76 L77
  constraint coincident A38 L78.end
  constraint perpendicular L75 L78
  constraint coincident L12 L79.start
  constraint perpendicular L12 L79
  constraint coincident A37 L80.end
  constraint perpendicular L79 L80
  constraint coincident A38 L81.end
  constraint perpendicular L79 L81
  constraint parallel L81 L82
  constraint coincident A30.centre L83.start
  constraint coincident L28 L83.end
  constraint perpendicular L28 L83
  constraint perpendicular L28 L84
  constraint coincident A37 L85.end
  constraint perpendicular L84 L85
  constraint perpendicular L54 L86
  constraint coincident L27.end L28.start
  constraint perpendicular L86 L87
  constraint coincident L53 L88.start
  constraint perpendicular L53 L88
  constraint perpendicular L87 L89
  constraint coincident L89 L90.end
  constraint perpendicular L89 L90
  constraint coincident A38 L91.end
  constraint perpendicular L88 L91
  constraint coincident A28.centre L92.start
  constraint perpendicular L40 L92
  constraint coincident A37 L93.end
  constraint perpendicular L92 L93
  constraint coincident L39.end L40.start
  constraint perpendicular L40 L94
  constraint coincident L94 L95.end
  constraint perpendicular L94 L95
  constraint coincident L56 L96.start
  constraint perpendicular L56 L96
  constraint coincident L94 L97.end
  constraint perpendicular L94 L97
  constraint coincident A38 L98.end
  constraint perpendicular L96 L98
  constraint coincident L26.end L27.start
  constraint perpendicular L26 L99
  constraint coincident L55 L100.start
  constraint perpendicular L55 L100
  constraint coincident L99 L101.end
  constraint perpendicular L99 L101
  constraint coincident A38 L102.end
  constraint perpendicular L100 L102
  constraint coincident A29.centre L103.start
  constraint perpendicular L26 L103
  constraint coincident L99 L104.end
  constraint perpendicular L99 L104
  constraint coincident A37 L105.end
  constraint perpendicular L103 L105
  constraint coincident L5 L106.start
  constraint perpendicular L5 L106
  constraint coincident A37 L107.end
  constraint perpendicular L106 L107
  constraint coincident A38 L108.end
  constraint perpendicular L106 L108
  constraint coincident L4 L109.start
  constraint perpendicular L4 L109
  constraint coincident A37 L110.end
  constraint perpendicular L109 L110
  constraint perpendicular L109 L111
  measures "d120" distance of A27.centre L71.end
  measures "d121" distance of L75.start L75.end
  measures "d122" distance of A30.centre L84.end
  measures "d123" distance of L88.start L88.end
  measures "d124" distance of A28.centre L92.end
  measures "d125" distance of L96.start L96.end
  measures "d126" distance of L100.start L100.end
  measures "d127" distance of A29.centre L103.end
extrude "押し出し27" cut sketch "スケッチ28" against normal blind 30 contours A37 A38 L80 L81 L85 L86 L87 L89 L90 L91 | A37 A38 L99 L101 L102 L104 L105 L107 L108 | A37 A38 L93 L94 L95 L97 L98 L110 L111 | A37 A38 L67 L68 L72 L73 L74 L76 L77 L78 bodies 1
sketch "スケッチ29" plane through (0, 0, 3) normal (0, 0, 1) x (-1, 0, 0)
  line L0 (28.5671, 78.0646) -> (41.4718, 65.1599)
  line L1 (41.4718, 65.1599) -> (21.4684, 45.1565)
  arc A0 (21.4684, 45.1565) -> (9, 49.1833) centre (0, 0) ccw
  line L2 (9, 49.1833) -> (9, 98.5901)
  arc A1 (40.7341, 90.2316) -> (9, 98.5901) centre (0, 0) ccw
  line L3 (40.7341, 90.2316) -> (28.5671, 78.0646)
  arc A2 (-9, 98.5901) -> (-40.7341, 90.2316) centre (0, 0) ccw
  line L4 (-9, 98.5901) -> (-9, 49.1833)
  arc A3 (-9, 49.1833) -> (-21.4684, 45.1565) centre (0, 0) ccw
  line L5 (-21.4684, 45.1565) -> (-41.4718, 65.1599)
  line L6 (-41.4718, 65.1599) -> (-28.5671, 78.0646)
  line L7 (-28.5671, 78.0646) -> (-40.7341, 90.2316)
  arc A4 (49.1833, 9) -> (45.1565, 21.4684) centre (0, 0) ccw
  line L8 (45.1565, 21.4684) -> (65.1599, 41.4718)
  line L9 (65.1599, 41.4718) -> (78.0646, 28.5671)
  line L10 (78.0646, 28.5671) -> (90.2316, 40.7341)
  arc A5 (98.5901, 9) -> (90.2316, 40.7341) centre (0, 0) ccw
  line L11 (98.5901, 9) -> (49.1833, 9)
  line L12 (-78.0646, 28.5671) -> (-65.1599, 41.4718)
  line L13 (-65.1599, 41.4718) -> (-45.1565, 21.4684)
  arc A6 (-45.1565, 21.4684) -> (-49.1833, 9) centre (0, 0) ccw
  line L14 (-49.1833, 9) -> (-98.5901, 9)
  arc A7 (-90.2316, 40.7341) -> (-98.5901, 9) centre (0, 0) ccw
  line L15 (-90.2316, 40.7341) -> (-78.0646, 28.5671)
  arc A8 (97.6998, -15.9925) -> (98.5884, -9.0182) centre (0, 0) ccw
  line L16 (97.6998, -15.9925) -> (85.6199, -9.0182)
  line L17 (85.6199, -9.0182) -> (98.5884, -9.0182)
  line L18 (-98.5884, -9.0182) -> (-85.6199, -9.0182)
  line L19 (-85.6199, -9.0182) -> (-97.6998, -15.9925)
  arc A9 (-98.5884, -9.0182) -> (-97.6998, -15.9925) centre (0, 0) ccw
  arc A10 (-4, 44.8219) -> (-30.0029, 33.5384) centre (0, 0) ccw
  line L20 (-4, 44.8219) -> (-4, 98.9192)
  arc A11 (4, 98.9192) -> (-4, 98.9192) centre (0, 0) ccw
  line L21 (4, 98.9192) -> (4, 44.8219)
  arc A12 (30.0029, 33.5384) -> (4, 44.8219) centre (0, 0) ccw
  line L22 (30.0029, 33.5384) -> (24.3354, 27.8709)
  arc A13 (24.3354, 27.8709) -> (-24.3354, 27.8709) centre (0, 0) ccw
  line L23 (-24.3354, 27.8709) -> (-30.0029, 33.5384)
  arc A14 (-44.8219, -4) -> (-33.5384, -30.0029) centre (0, 0) ccw
  line L24 (-44.8219, -4) -> (-98.9192, -4)
  arc A15 (-98.9192, 4) -> (-98.9192, -4) centre (0, 0) ccw
  line L25 (-98.9192, 4) -> (-44.8219, 4)
  arc A16 (-33.5056, 30.0396) -> (-44.8219, 4) centre (0, 0) ccw
  line L26 (-33.5056, 30.0396) -> (-27.9198, 24.2793)
  arc A17 (-27.9198, 24.2793) -> (-27.8709, -24.3354) centre (0, 0) ccw
  line L27 (-27.8709, -24.3354) -> (-33.5384, -30.0029)
  arc A18 (44.8219, 4) -> (33.5384, 30.0029) centre (0, 0) ccw
  line L28 (44.8219, 4) -> (98.9192, 4)
  arc A19 (98.9192, -4) -> (98.9192, 4) centre (0, 0) ccw
  line L29 (98.9192, -4) -> (44.8219, -4)
  arc A20 (33.5384, -30.0029) -> (44.8219, -4) centre (0, 0) ccw
  line L30 (33.5384, -30.0029) -> (27.8709, -24.3354)
  arc A21 (27.8709, -24.3354) -> (27.8709, 24.3354) centre (0, 0) ccw
  line L31 (27.8709, 24.3354) -> (33.5384, 30.0029)
  arc A22 (4, -44.8219) -> (30.0029, -33.5384) centre (0, 0) ccw
  line L32 (4, -44.8219) -> (4, -50)
  line L33 (4, -50) -> (40, -50)
  line L34 (40, -50) -> (40, -58)
  line L35 (40, -58) -> (-40, -58)
  line L36 (-40, -58) -> (-40, -50)
  line L37 (-40, -50) -> (-4, -50)
  line L38 (-4, -50) -> (-4, -47)
  line L39 (-4, -47) -> (-4, -44.8219)
  arc A23 (-30.0678, -33.4802) -> (-4, -44.8219) centre (0, 0) ccw
  line L40 (-30.0678, -33.4802) -> (-24.308, -27.8949)
  arc A24 (-24.308, -27.8949) -> (24.3354, -27.8709) centre (0, 0) ccw
  line L41 (24.3354, -27.8709) -> (30.0029, -33.5384)
  line L42 (26.0567, 42.6737) -> (45.0073, 61.6244)
  line L43 (45.0073, 61.6244) -> (61.6244, 45.0073)
  line L44 (61.6244, 45.0073) -> (42.6737, 26.0567)
  arc A25 (42.6737, 26.0567) -> (26.0567, 42.6737) centre (0, 0) ccw
  line L45 (-36.2136, -34.4757) -> (-59.4233, -47.8758)
  line L46 (-59.4233, -47.8758) -> (-71.1733, -27.5242)
  line L47 (-71.1733, -27.5242) -> (-47.9636, -14.1241)
  arc A26 (-47.9636, -14.1241) -> (-36.2136, -34.4757) centre (0, 0) ccw
  arc A27 (-32.4242, -38.0614) -> (-21.7945, -45) centre (0, 0) ccw
  line L48 (-21.7945, -45) -> (-44.4423, -45)
  line L49 (-44.4423, -45) -> (-32.4242, -38.0614)
  line L50 (81.8683, -9) -> (73.6733, -23.1941)
  line L51 (73.6733, -23.1941) -> (49.1742, -9.0495)
  line L52 (49.1742, -9.0495) -> (75, -9)
  line L53 (75, -9) -> (81.8683, -9)
  line L54 (-42.6737, 26.0567) -> (-61.6244, 45.0073)
  line L55 (-61.6244, 45.0073) -> (-45.0073, 61.6244)
  line L56 (-45.0073, 61.6244) -> (-26.0567, 42.6737)
  arc A28 (-26.0567, 42.6737) -> (-42.6737, 26.0567) centre (0, 0) ccw
  line L57 (47.9636, -14.1241) -> (71.1733, -27.5242)
  line L58 (71.1733, -27.5242) -> (59.4233, -47.8758)
  line L59 (59.4233, -47.8758) -> (36.2136, -34.4757)
  arc A29 (36.2136, -34.4757) -> (47.9636, -14.1241) centre (0, 0) ccw
  line L60 (-81.8759, -8.9868) -> (-49.1742, -9.0495)
  line L61 (-49.1742, -9.0495) -> (-73.6733, -23.1941)
  line L62 (-73.6733, -23.1941) -> (-81.8759, -8.9868)
  line L63 (32.4242, -38.0614) -> (44.4423, -45)
  line L64 (44.4423, -45) -> (21.7945, -45)
  arc A30 (21.7945, -45) -> (32.4242, -38.0614) centre (0, 0) ccw
  circle A31 centre (0, 0) radius 32
  circle A32 centre (-51.2451, -46.0409) radius 1.5
  circle A33 centre (51.2451, -46.0409) radius 1.5
  circle A34 centre (-65.4951, -21.3591) radius 1.5
  circle A35 centre (-57.7353, 37.5827) radius 1.5
  circle A36 centre (-37.5827, 57.7353) radius 1.5
  circle A37 centre (37.5827, 57.7353) radius 1.5
  circle A38 centre (57.7353, 37.5827) radius 1.5
  circle A39 centre (65.4951, -21.3591) radius 1.5
  line L65 (40, -84.2208) -> (61.0153, -84.2208)
  arc A40 (61.0153, -84.2208) -> (71.238, -75.7703) centre (0, 0) ccw
  line L66 (71.238, -75.7703) -> (54.6284, -66.1808)
  line L67 (54.6284, -66.1808) -> (84.6284, -14.2192)
  line L68 (84.6284, -14.2192) -> (101.238, -23.8088)
  arc A41 (101.238, -23.8088) -> (91.6263, 49.1999) centre (0, 0) ccw
  line L69 (91.6263, 49.1999) -> (78.0646, 35.6382)
  line L70 (78.0646, 35.6382) -> (35.6382, 78.0646)
  line L71 (35.6382, 78.0646) -> (49.1999, 91.6263)
  arc A42 (49.1999, 91.6263) -> (-49.1999, 91.6263) centre (0, 0) ccw
  line L72 (-49.1999, 91.6263) -> (-35.6382, 78.0646)
  line L73 (-35.6382, 78.0646) -> (-78.0646, 35.6382)
  line L74 (-78.0646, 35.6382) -> (-91.6263, 49.1999)
  arc A43 (-91.6263, 49.1999) -> (-101.238, -23.8088) centre (0, 0) ccw
  line L75 (-101.238, -23.8088) -> (-84.6284, -14.2192)
  line L76 (-84.6284, -14.2192) -> (-54.6284, -66.1808)
  line L77 (-54.6284, -66.1808) -> (-71.238, -75.7703)
  arc A44 (-71.238, -75.7703) -> (-61.3188, -84) centre (0, 0) ccw
  line L78 (-61.3188, -84) -> (-40, -84)
  line L79 (-40, -84) -> (-40, -64)
  line L80 (-40, -64) -> (40, -64)
  line L81 (40, -64) -> (40, -84.2208)
  line L82 (-44.4423, -45) -> (-61.2534, -54.7059)
  line L83 (-57.7592, -60.7582) -> (-53.429, -58.2582)
  line L84 (-53.429, -58.2582) -> (-56.9233, -52.2059)
  line L85 (-50.114, -64) -> (-53.429, -58.2582)
  line L86 (-45, -50.5) -> (-45, -50)
  line L87 (-45, -50) -> (-53.1025, -50)
  line L88 (-45, -50.5) -> (-45, -64)
  line L89 (-45, -64) -> (-50.114, -64)
  line L90 (44.4423, -45) -> (61.2534, -54.7059)
  line L91 (58.1185, -60.1358) -> (53.7884, -57.6358)
  line L92 (53.7884, -57.6358) -> (56.9233, -52.2059)
  line L93 (40, -64) -> (45, -64)
  line L94 (45, -64) -> (51, -64)
  line L95 (53.7884, -57.6358) -> (50.114, -64)
  line L96 (45, -64) -> (45, -50)
  line L97 (45, -50) -> (52.8479, -49.853)
  dimension "d130" = 5
  dimension "d131" = 5
  constraint coincident L48.end L49.start
  constraint coincident L76 L82.end
  constraint perpendicular L76 L82
  constraint coincident L76 L83.start
  constraint perpendicular L76 L83
  constraint coincident L82 L84.end
  constraint perpendicular L82 L84
  constraint perpendicular L83 L85
  constraint vertical L86
  constraint coincident L82 L87.end
  constraint perpendicular L86 L87
  constraint perpendicular L87 L88
  constraint coincident L63.end L64.start
  constraint coincident L67 L90.end
  constraint perpendicular L67 L90
  constraint coincident L67 L91.start
  constraint perpendicular L67 L91
  constraint coincident L90 L92.end
  constraint perpendicular L90 L92
  constraint coincident L80.end L81.start
  constraint perpendicular L81 L93
  constraint perpendicular L81 L94
  constraint coincident L94 L95.end
  constraint perpendicular L91 L95
  constraint perpendicular L93 L96
  constraint midpoint L90 L97.end
  measures "d130" distance of L83.start L83.end
  measures "d131" distance of L91.start L91.end
extrude "押し出し28" cut sketch "スケッチ29" against normal blind 45 contours L90 L92 L94 L95 L96 L97 | L82 L84 L85 L86 L87 L88 L89 bodies 1
fillet "フィレット1" radius 2 6 edges at (32.4242, 38.0614, 2.25) (-32.4242, 38.0614, 2.25) (44.4423, 45, 2.25) (-21.7945, 45, 2.25) (-44.4423, 45, 2.25) (21.7945, 45, 2.25) on bodies 1
fillet "フィレット2" radius 2 5 edges at (-45, 64, 2.25) (-50.114, 64, 2.25) (-52.8479, 49.853, 2.25) (-45, 50, 2.25) (-56.9233, 52.2059, 2.25) on bodies 1
fillet "フィレット3" radius 2 5 edges at (45, 50, 2.25) (53.1025, 50, 2.25) (56.9233, 52.2059, 2.25) (50.114, 64, 2.25) (45, 64, 2.25) on bodies 1
fillet "フィレット4" radius 2 6 edges at (85.6199, 9.0182, 2.25) (98.5884, 9.0182, 2.25) (97.6998, 15.9925, 2.25) (-97.6998, 15.9925, 2.25) (-98.5884, 9.0182, 2.25) (-85.6199, 9.0182, 2.25) on bodies 1
fillet "フィレット5" radius 2 3 edges at (-49.1742, 9.0495, 2.25) (-73.6733, 23.1941, 2.25) (-81.8683, 9, 2.25) on bodies 1
fillet "フィレット6" radius 2 3 edges at (49.1742, 9.0495, 2.25) (81.8759, 8.9868, 2.25) (73.6733, 23.1941, 2.25) on bodies 1
fillet "フィレット7" radius 2 4 edges at (71.1733, 27.5242, 2.25) (59.4233, 47.8758, 2.25) (36.2136, 34.4757, 2.25) (47.9636, 14.1241, 2.25) on bodies 1
fillet "フィレット8" radius 2 4 edges at (-36.2136, 34.4757, 2.25) (-47.9636, 14.1241, 2.25) (-59.4233, 47.8758, 2.25) (-71.1733, 27.5242, 2.25) on bodies 1
fillet "フィレット9" radius 2 8 edges at (-40, 50, 2.25) (-4, 50, 2.25) (-4, 44.8219, 2.25) (4, 50, 2.25) (4, 44.8219, 2.25) (40, 50, 2.25) (40, 58, 2.25) (-40, 58, 2.25) on bodies 1
fillet "フィレット10" radius 2 4 edges at (-24.3354, 27.8709, 2.25) (24.308, 27.8949, 2.25) (30.0678, 33.4802, 2.25) (-30.0029, 33.5384, 2.25) on bodies 1
fillet "フィレット11" radius 2 8 edges at (-98.9192, -4, 2.25) (-44.8219, -4, 2.25) (-44.8219, 4, 2.25) (-98.9192, 4, 2.25) (98.9192, 4, 2.25) (98.9192, -4, 2.25) (44.8219, -4, 2.25) (44.8219, 4, 2.25) on bodies 1
fillet "フィレット12" radius 2 6 edges at (-98.5901, -9, 2.25) (-90.2316, -40.7341, 2.25) (-78.0646, -28.5671, 2.25) (-65.1599, -41.4718, 2.25) (-45.1565, -21.4684, 2.25) (-49.1833, -9, 2.25) on bodies 1
fillet "フィレット13" radius 2 6 edges at (98.5901, -9, 2.25) (78.0646, -28.5671, 2.25) (90.2316, -40.7341, 2.25) (65.1599, -41.4718, 2.25) (49.1833, -9, 2.25) (45.1565, -21.4684, 2.25) on bodies 1
fillet "フィレット14" radius 2 4 edges at (26.0567, -42.6737, 2.25) (42.6737, -26.0567, 2.25) (45.0073, -61.6244, 2.25) (61.6244, -45.0073, 2.25) on bodies 1
fillet "フィレット15" radius 2 4 edges at (-26.0567, -42.6737, 2.25) (-42.6737, -26.0567, 2.25) (-61.6244, -45.0073, 2.25) (-45.0073, -61.6244, 2.25) on bodies 1
fillet "フィレット16" radius 2 4 edges at (-27.8709, -24.3354, 2.25) (-27.8709, 24.3354, 2.25) (-33.5384, 30.0029, 2.25) (-33.5384, -30.0029, 2.25) on bodies 1
fillet "フィレット17" radius 2 4 edges at (33.5056, -30.0396, 2.25) (27.9198, -24.2793, 2.25) (27.8709, 24.3354, 2.25) (33.5384, 30.0029, 2.25) on bodies 1
fillet "フィレット18" radius 2 6 edges at (24.3354, -27.8709, 2.25) (-24.3354, -27.8709, 2.25) (30.0029, -33.5384, 2.25) (-30.0029, -33.5384, 2.25) (-4, -44.8219, 2.25) (4, -44.8219, 2.25) on bodies 1
fillet "フィレット19" radius 2 3 edges at (-40.7341, -90.2316, 2.25) (-28.5671, -78.0646, 2.25) (-41.4718, -65.1599, 2.25) on bodies 1
fillet "フィレット20" radius 2 3 edges at (40.7341, -90.2316, 2.25) (28.5671, -78.0646, 2.25) (41.4718, -65.1599, 2.25) on bodies 1
fillet "フィレット21" radius 2 8 edges at (-9, -98.5901, 2.25) (-9, -49.1833, 2.25) (-21.4684, -45.1565, 2.25) (9, -49.1833, 2.25) (9, -98.5901, 2.25) (-4, -98.9192, 2.25) (4, -98.9192, 2.25) (21.4684, -45.1565, 2.25) on bodies 1
delete_face "面を削除1" 1 faces at (-29.8533, -79.338, 2) on bodies 1
delete_face "面を削除2" 1 faces at (29.7392, -76.9436, 2) on bodies 1
fillet "フィレット22" radius 4 2 edges at (28.5671, -78.0646, 2.25) (-28.5671, -78.0646, 2.25) on bodies 1
fillet "フィレット23" radius 2 2 edges at (35.6382, -78.0646, 2.25) (78.0646, -35.6382, 2.25) on bodies 1
delete_face "面を削除3" 1 faces at (79.1856, -29.7392, 2) on bodies 1
fillet "フィレット24" radius 4 1 edges at (78.0646, -28.5671, 2.25) on bodies 1
fillet "フィレット25" radius 4 2 edges at (91.6263, -49.1999, 2.25) (49.1999, -91.6263, 2.25) on bodies 1
fillet "フィレット26" radius 4 2 edges at (-91.6263, -49.1999, 2.25) (-49.1999, -91.6263, 2.25) on bodies 1
fillet "フィレット27" radius 2 2 edges at (-35.6382, -78.0646, 2.25) (-78.0646, -35.6382, 2.25) on bodies 1
fillet "フィレット28" radius 2 6 edges at (-84.6284, 14.2192, 2.25) (-54.6284, 66.1808, 2.25) (-40, 64, 2.25) (84.6284, 14.2192, 2.25) (40, 64, 2.25) (54.6284, 66.1808, 2.25) on bodies 1
fillet "フィレット29" radius 4 4 edges at (101.238, 23.8088, 2.25) (71.238, 75.7703, 2.25) (-101.238, 23.8088, 2.25) (-71.238, 75.7703, 2.25) on bodies 1
fillet "フィレット30" radius 4 2 edges at (40, 84, 2.25) (-40, 84.2208, 2.25) on bodies 1